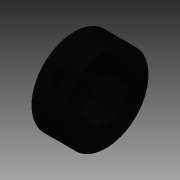
# Autodesk Inventor part: Hex Shaft Collar
Saved by Autodesk Inventor 2015 (Build 190159000, 159)
## iProperties
Created: 2014-06-25
Part Number: Hex Shaft Collar
Material: Aluminum 6061
Document SubType Name: Modeling
Designer: Evan
Density: 2.7 g/cm^3
Appearance: Anodized - Black
Author: Evan
Autodesk Inventor part; units mm, degrees
ref_plane "YZ Plane" through (0, 0, 0) normal (1, 0, 0) x (0, 1, 0)
ref_plane "XZ Plane" through (0, 0, 0) normal (0, 1, 0) x (-1, 0, 0)
sketch "Sketch1" plane through (0, 0, 0) normal (1, 0, 0) x (0, 1, 0)
  line L0 (0, -7.0612) -> (-6.1152, -3.5306)
  line L1 (-6.1152, -3.5306) -> (-6.1152, 3.5306)
  line L2 (-6.1152, 3.5306) -> (0, 7.0612)
  line L3 (0, 7.0612) -> (6.1152, 3.5306)
  line L4 (6.1152, 3.5306) -> (6.1152, -3.5306)
  line L5 (6.1152, -3.5306) -> (0, -7.0612)
  circle A0 centre (0, 0) radius 12.7
  dimension "d0" = 7.0612
  dimension "d1" = 25.4
  constraints: 12 end point, 2 coincident, 1 centre point, 13 other
  measures "d0" distance of L3.end L4.end
  measures "d1" diameter of A0
extrude "Extrusion1" add sketch "Sketch1" along normal blind 9.525
ref_plane "Work Plane1" through (0, 12.7, 0) normal (0, -1, 0) x (1, 0, 0)
sketch "Sketch2" plane through (0, 12.7, 0) normal (0, -1, 0) x (1, 0, 0)
  circle A0 centre (4.7625, 9.652) radius 1.524
  circle A1 centre (4.7625, -9.652) radius 1.524
  line L0 (0, 12.7) -> (0, -12.7) projected
  point P0 (0, 0)
  dimension "d4" = 3.048
  dimension "d5" = 3.048
  dimension "d6" = 4.7625
  dimension "d7" = 4.7625
  dimension "d8" = 9.652
  dimension "d9" = 9.652
  constraints: 2 centre point
  measures "d4" diameter of A0
  measures "d5" diameter of A1
  measures "d6" distance from line of L0 A0.centre
  measures "d7" distance from line of L0 A1.centre
  measures "d8" vertical distance of point (0, 0) A0.centre
  measures "d9" vertical distance of point (0, 0) A1.centre
extrude "Extrusion2" cut sketch "Sketch2" along normal blind 25.4
body "Solid1"
